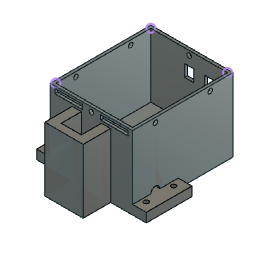
CircuitEnclosure (Autodesk Fusion 360 design; units mm, degrees)
Autodesk Fusion 360 part; units mm, degrees
sketch "Sketch1" plane through (0, 0, 0) normal (0, 1, 0) x (1, 0, 0)
  line L0 (0, 0) -> (60, 0)
  line L1 (60, 0) -> (-60, 0)
  line L2 (-60, 0) -> (-60, -50)
  line L3 (-60, -50) -> (60, -50)
  line L4 (60, -50) -> (60, 0)
  line L5 (-60, 0) -> (-45, 0)
  line L6 (60, 0) -> (45, 0)
  line L7 (-45, 0) -> (-45, 60)
  line L8 (45, 0) -> (45, 60)
  line L9 (-45, 60) -> (45, 60)
  dimension "d1" = 60
  dimension "d2" = 120
  dimension "d3" = 50
  dimension "d4" = 15
  dimension "d5" = 15
  dimension "d6" = 60
  dimension "d7" = 60
  constraint coincident L0.start origin
  constraint horizontal L0
  constraint parallel L0 L1
  constraint perpendicular L1 L2
  constraint perpendicular L2 L3
  constraint perpendicular L1 L4
  constraint perpendicular L2 L5
  constraint perpendicular L4 L6
  constraint perpendicular L5 L7
  constraint perpendicular L6 L8
  measures "d1" distance of L0.start L0.end
  measures "d2" distance of L0.end L1.end
  measures "d3" distance of L1.end L2.end
  measures "d4" distance of L1.end L5.end
  measures "d5" distance of L0.end L6.end
  measures "d6" distance of L5.end L7.end
  measures "d7" distance of L6.end L8.end
extrude "Extrude1" add sketch "Sketch1" along normal blind 10
sketch "Sketch2" plane through (0, 10, 0) normal (0, 1, 0) x (-1, 0, 0)
  line L0 (60, 0) -> (60, 50)
  line L1 (60, 50) -> (-60, 50)
  line L2 (-60, 50) -> (-60, 0)
  line L3 (-60, 0) -> (-45, 0)
  line L4 (-45, 0) -> (-45, -60)
  line L5 (-45, -60) -> (45, -60)
  line L6 (45, -60) -> (45, 0)
  line L7 (45, 0) -> (60, 0)
  line L8 (60, 50) -> (60, 40)
  line L9 (-60, 50) -> (-60, 40)
  circle A0 centre (50, 40) radius 2.5
  circle A1 centre (-50, 40) radius 2.5
  circle A2 centre (50, 10) radius 2.5
  circle A3 centre (-50, 10) radius 2.5
  dimension "d10" = 10
  dimension "d11" = 10
  dimension "d12" = 10
  dimension "d13" = 10
  dimension "d14" = 5
  dimension "d15" = 5
  dimension "d16" = 30
  dimension "d17" = 5
  dimension "d18" = 30
  dimension "d19" = 5
  constraint coincident L0.end L1.start
  constraint perpendicular L1 L8
  constraint coincident L1.end L2.start
  constraint perpendicular L1 L9
  measures "d10" distance of L0.end L8.end
  measures "d11" distance of L8.end A0.centre
  measures "d12" distance of L1.end L9.end
  measures "d13" distance of L9.end A1.centre
  measures "d14" diameter of A0
  measures "d15" diameter of A1
  measures "d16" distance of A0.centre A2.centre
  measures "d17" diameter of A2
  measures "d18" distance of A1.centre A3.centre
  measures "d19" diameter of A3
extrude "Extrude2" cut sketch "Sketch2" against normal blind 20 contours A0 | A1 | A2 | A3
sketch "Sketch3" plane through (0, 10, 0) normal (0, 1, 0) x (-1, 0, 0)
  circle A0 centre (50, 40) radius 2.5
  circle A1 centre (-50, 40) radius 2.5
  circle A2 centre (50, 10) radius 2.5
  circle A3 centre (-50, 10) radius 2.5
  line L0 (60, 0) -> (60, 50)
  line L1 (60, 50) -> (-60, 50)
  line L2 (-60, 50) -> (-60, 0)
  line L3 (-60, 0) -> (-45, 0)
  line L4 (-45, 0) -> (-45, -60)
  line L5 (-45, -60) -> (45, -60)
  line L6 (45, -60) -> (45, 0)
  line L7 (45, 0) -> (60, 0)
  line L8 (45, -60) -> (45, 50)
  line L9 (-45, -60) -> (-45, 50)
  line L10 (45, 50) -> (-45, 50)
  line L11 (-45, -60) -> (45, -60)
  line L12 (45, 50) -> (42, 50)
  line L13 (45, -60) -> (42, -60)
  line L14 (-45, -60) -> (-45, -57)
  line L15 (-45, 50) -> (-42, 50)
  line L16 (42, 47) -> (42, -57)
  line L17 (-42, -57) -> (42, -57)
  line L18 (-42, -57) -> (-42, 47)
  line L19 (-42, 47) -> (42, 47)
  dimension "d22" = 3
  dimension "d23" = 3
  dimension "d24" = 3
  dimension "d25" = 3
  dimension "d26" = 3
  dimension "d27" = 3
  dimension "d28" = 3
  dimension "d29" = 3
  constraint coincident L5.end L6.start
  constraint coincident L1 L8.end
  constraint perpendicular L1 L8
  constraint coincident L4.end L5.start
  constraint coincident L1 L9.end
  constraint perpendicular L1 L9
  constraint perpendicular L8 L12
  constraint perpendicular L6 L13
  constraint perpendicular L11 L14
  constraint perpendicular L9 L15
  measures "d22" distance of L8.end L12.end
  measures "d23" distance of L12.end L16.start
  measures "d24" distance of L5.end L13.end
  measures "d25" distance of L13.end L16.end
  measures "d26" distance of L4.end L14.end
  measures "d27" distance of L14.end L17.start
  measures "d28" distance of L9.end L15.end
  measures "d29" distance of L15.end L18.end
extrude "Extrude3" add sketch "Sketch3" along normal blind 70 contours L1 L4 L5 L6 L8 L9 L10 L11 L12 L13 L14 L15
sketch "Sketch4" plane through (-45, 0, 0) normal (-1, 0, 0) x (0, 0, 1)
  line L0 (-60, 0) -> (0, 0)
  line L1 (0, 0) -> (0, 10)
  line L2 (0, 10) -> (50, 10)
  line L3 (50, 10) -> (50, 80)
  line L4 (50, 80) -> (-60, 80)
  line L5 (-60, 80) -> (-60, 0)
  line L6 (-60, 80) -> (-60, 75)
  circle A0 centre (-35, 75) radius 2.5
  circle A1 centre (25, 75) radius 2.5
  dimension "d32" = 25
  dimension "d34" = 5
  dimension "d35" = 5
  constraint coincident L4.end L5.start
  constraint coincident L5 L6.end
  constraint perpendicular L4 L6
  measures "d32" distance of L6.end A0.centre
  measures "d34" diameter of A0
  measures "d35" diameter of A1
extrude "Extrude4" cut sketch "Sketch4" against normal blind 10 contours A0 | A1
sketch "Sketch5" plane through (45, 0, 0) normal (1, 0, 0) x (0, 0, -1)
  line L0 (0, 0) -> (60, 0)
  line L1 (60, 0) -> (60, 80)
  line L2 (60, 80) -> (-50, 80)
  line L3 (-50, 80) -> (-50, 10)
  line L4 (-50, 10) -> (0, 10)
  line L5 (0, 10) -> (0, 0)
  line L6 (-50, 80) -> (-50, 75)
  circle A0 centre (-25, 75) radius 2.5
  circle A1 centre (35, 75) radius 2.5
  dimension "d38" = 5
  dimension "d39" = 25
  dimension "d41" = 5
  dimension "d42" = 5
  constraint coincident L2.end L3.start
  constraint perpendicular L2 L6
  measures "d38" distance of L2.end L6.end
  measures "d39" distance of L6.end A0.centre
  measures "d41" diameter of A0
  measures "d42" diameter of A1
extrude "Extrude5" cut sketch "Sketch5" against normal blind 11 contours A0 | A1
sketch "Sketch6" plane through (0, 0, 50) normal (0, 0, 1) x (1, 0, 0)
  line L0 (-60, 0) -> (60, 0)
  line L1 (60, 0) -> (60, 10)
  line L2 (60, 10) -> (45, 10)
  line L3 (45, 10) -> (45, 80)
  line L4 (45, 80) -> (-45, 80)
  line L5 (-45, 80) -> (-45, 10)
  line L6 (-45, 10) -> (-60, 10)
  line L7 (-60, 10) -> (-60, 0)
  circle A0 centre (0, 75) radius 2.5
  dimension "d47" = 5
  measures "d47" diameter of A0
extrude "Extrude6" cut sketch "Sketch6" against normal blind 11 contours A0
sketch "Sketch7" plane through (0, 0, -60) normal (0, 0, -1) x (-1, 0, 0)
  line L0 (-45, 0) -> (45, 0)
  line L1 (45, 0) -> (45, 80)
  line L2 (45, 80) -> (-45, 80)
  line L3 (-45, 80) -> (-45, 0)
  circle A0 centre (0, 75) radius 2.5
  dimension "d51" = 5
  measures "d51" diameter of A0
extrude "Extrude7" cut sketch "Sketch7" against normal blind 11 contours A0
sketch "Sketch8" plane through (0, 0, 50) normal (0, 0, 1) x (1, 0, 0)
  circle A0 centre (0, 75) radius 2.5
  line L0 (-60, 0) -> (60, 0)
  line L1 (60, 0) -> (60, 10)
  line L2 (60, 10) -> (45, 10)
  line L3 (45, 10) -> (45, 80)
  line L4 (45, 80) -> (-45, 80)
  line L5 (-45, 80) -> (-45, 10)
  line L6 (-45, 10) -> (-60, 10)
  line L7 (-60, 10) -> (-60, 0)
  line L8 (-45, 80) -> (-45, 75)
  line L9 (-15, 77.5) -> (-35, 77.5)
  line L10 (-35, 72.5) -> (-15, 72.5)
  line L11 (-15, 77.5) -> (-10, 77.5)
  line L12 (-10, 77.5) -> (-10, 72.5)
  line L13 (-10, 72.5) -> (-15, 72.5)
  line L14 (-35, 77.5) -> (-40, 77.5)
  line L15 (-40, 77.5) -> (-40, 72.5)
  line L16 (-40, 72.5) -> (-35, 72.5)
  dimension "d55" = 20
  dimension "d56" = 5
  dimension "d57" = 5
  constraint coincident L4.end L5.start
  constraint coincident L5 L8.end
  constraint perpendicular L4 L8
  constraint perpendicular L11 L12
  constraint perpendicular L14 L15
  measures "d55" distance of L9.start L9.end
  measures "d56" distance of L9.end L10.start
  measures "d57" distance of L11.end L12.end
extrude "Extrude8" cut sketch "Sketch8" against normal blind 20 contours L9 L10 L11 L12 L13 L14 L15 L16
sketch "Sketch9" plane through (0, 0, 50) normal (0, 0, 1) x (1, 0, 0)
  line L0 (-40, 72.5) -> (-40, 77.5)
  line L1 (-40, 77.5) -> (-10, 77.5)
  line L2 (-10, 77.5) -> (-10, 72.5)
  line L3 (-10, 72.5) -> (-40, 72.5)
  circle A0 centre (0, 75) radius 2.5
  line L4 (-60, 0) -> (60, 0)
  line L5 (60, 0) -> (60, 10)
  line L6 (60, 10) -> (45, 10)
  line L7 (45, 10) -> (45, 80)
  line L8 (45, 80) -> (-45, 80)
  line L9 (-45, 80) -> (-45, 10)
  line L10 (-45, 10) -> (-60, 10)
  line L11 (-60, 10) -> (-60, 0)
  line L12 (45, 80) -> (45, 75)
  line L13 (45, 75) -> (40, 75)
  line L14 (40, 75) -> (40, 72.5)
  line L15 (40, 75) -> (40, 77.5)
  line L16 (40, 77.5) -> (10, 77.5)
  line L17 (10, 77.5) -> (10, 72.5)
  line L18 (10, 72.5) -> (40, 72.5)
  dimension "d60" = 2.5
  dimension "d61" = 2.5
  dimension "d62" = 30
  dimension "d63" = 5
  constraint coincident L7.end L8.start
  constraint coincident L7 L12.end
  constraint perpendicular L8 L12
  constraint perpendicular L12 L13
  constraint perpendicular L13 L14
  constraint perpendicular L13 L15
  constraint perpendicular L15 L16
  constraint perpendicular L16 L17
  measures "d60" distance of L13.end L14.end
  measures "d61" distance of L13.end L15.end
  measures "d62" distance of L15.end L16.end
  measures "d63" distance of L16.end L17.end
extrude "Extrude9" cut sketch "Sketch9" against normal blind 20 contours L14 L15 L16 L17 L18
sketch "Sketch10" plane through (0, 0, 0) normal (0, -1, 0) x (1, 0, 0)
  circle A0 centre (-50, 40) radius 2.5
  circle A1 centre (50, 40) radius 2.5
  circle A2 centre (-50, 10) radius 2.5
  circle A3 centre (50, 10) radius 2.5
  line L0 (-60, 50) -> (-60, 0)
  line L1 (-60, 0) -> (-45, 0)
  line L2 (-45, 0) -> (-45, -60)
  line L3 (-45, -60) -> (45, -60)
  line L4 (45, -60) -> (45, 0)
  line L5 (45, 0) -> (60, 0)
  line L6 (60, 0) -> (60, 50)
  line L7 (60, 50) -> (-60, 50)
  line L8 (0, 50) -> (11, 50)
  line L9 (11, 50) -> (11, 72)
  line L10 (11, 72) -> (-11, 72)
  line L11 (-11, 72) -> (-11, 50)
  line L12 (-11, 50) -> (-21, 50)
  line L13 (-21, 50) -> (-21, 80)
  line L14 (-21, 80) -> (21, 80)
  line L15 (21, 80) -> (21, 50)
  dimension "d66" = 11
  dimension "d67" = 22
  dimension "d68" = 22
  dimension "d69" = 10
  constraint midpoint L7 L8.start
  constraint parallel L7 L8
  constraint perpendicular L8 L9
  constraint perpendicular L9 L10
  constraint coincident L7 L11.end
  constraint perpendicular L7 L11
  constraint perpendicular L11 L12
  constraint perpendicular L7 L13
  constraint perpendicular L13 L14
  constraint coincident L7 L15.end
  constraint perpendicular L7 L15
  measures "d66" distance of L8.start L8.end
  measures "d67" distance of L8.end L9.end
  measures "d68" distance of L9.end L10.end
  measures "d69" distance of L11.end L12.end
extrude "Extrude10" add sketch "Sketch10" against normal blind 70 contours L7 L9 L10 L11 L12 L13 L14 L15
sketch "Sketch11" plane through (0, 0, 0) normal (0, -1, 0) x (1, 0, 0)
  line L0 (-21, 50) -> (-60, 50)
  line L1 (-60, 50) -> (-60, 0)
  line L2 (-60, 0) -> (-45, 0)
  line L3 (-45, 0) -> (-45, -60)
  line L4 (-45, -60) -> (45, -60)
  line L5 (45, -60) -> (45, 0)
  line L6 (45, 0) -> (60, 0)
  line L7 (60, 0) -> (60, 50)
  line L8 (60, 50) -> (21, 50)
  line L9 (21, 50) -> (21, 80)
  line L10 (21, 80) -> (-21, 80)
  line L11 (-21, 80) -> (-21, 50)
  circle A0 centre (-50, 40) radius 2.5
  circle A1 centre (50, 40) radius 2.5
  circle A2 centre (-50, 10) radius 2.5
  circle A3 centre (50, 10) radius 2.5
  line L12 (-11, 50) -> (-11, 72)
  line L13 (-11, 72) -> (11, 72)
  line L14 (11, 72) -> (11, 50)
  line L15 (11, 50) -> (-11, 50)
sketch "Sketch12" plane through (0, 0, 0) normal (0, -1, 0) x (1, 0, 0)
sketch "Sketch13" plane through (0, 0, 80) normal (0, 0, 1) x (1, 0, 0)
  line L0 (-21, 0) -> (21, 0)
  line L1 (21, 0) -> (21, 70)
  line L2 (21, 70) -> (-21, 70)
  line L3 (-21, 70) -> (-21, 0)
sketch "Sketch14" plane through (-45, 0, 0) normal (-1, 0, 0) x (0, 0, 1)
  circle A0 centre (25, 75) radius 2.5
  circle A1 centre (-35, 75) radius 2.5
  line L0 (-60, 0) -> (0, 0)
  line L1 (0, 0) -> (0, 10)
  line L2 (0, 10) -> (50, 10)
  line L3 (50, 10) -> (50, 80)
  line L4 (50, 80) -> (-60, 80)
  line L5 (-60, 80) -> (-60, 0)
  line L6 (0, 10) -> (25, 10)
  arc A2 (30, 10) -> (20, 10) centre (25, 10) ccw
  dimension "d72" = 10
  constraint coincident L1.end L2.start
  constraint midpoint L2 L6.end
  constraint coincident L6.end A2.centre
  constraint coincident L2 A2.end
  constraint coincident L2 A2.start
  measures "d72" diameter of A2
extrude "Extrude11" cut sketch "Sketch14" against normal blind 100 contours L2 L6 A2
sketch "Sketch15" plane through (0, 0, -60) normal (0, 0, -1) x (-1, 0, 0)
  circle A0 centre (0, 75) radius 2.5
  line L0 (-45, 0) -> (45, 0)
  line L1 (45, 0) -> (45, 80)
  line L2 (45, 80) -> (-45, 80)
  line L3 (-45, 80) -> (-45, 0)
  line L4 (-45, 80) -> (-45, 65)
  line L5 (-30, 65) -> (-17, 65)
  line L6 (-30, 65) -> (-30, 47)
  line L7 (-30, 47) -> (-17, 47)
  line L8 (-17, 47) -> (-17, 65)
  dimension "d76" = 13
  dimension "d77" = 18
  dimension "d78" = 13
  constraint coincident L2.end L3.start
  constraint coincident L3 L4.end
  constraint perpendicular L3 L5
  constraint perpendicular L5 L6
  constraint perpendicular L6 L7
  measures "d76" distance of L5.start L5.end
  measures "d77" distance of L5.start L6.end
  measures "d78" distance of L6.end L7.end
extrude "Extrude12" cut sketch "Sketch15" against normal blind 20 contours L5 L6 L7 L8
sketch "Sketch16" plane through (0, 0, -60) normal (0, 0, -1) x (-1, 0, 0)
  line L0 (-17, 47) -> (-30, 47)
  line L1 (-30, 47) -> (-30, 65)
  line L2 (-30, 65) -> (-17, 65)
  line L3 (-17, 65) -> (-17, 47)
  circle A0 centre (0, 75) radius 2.5
  line L4 (-45, 0) -> (45, 0)
  line L5 (45, 0) -> (45, 80)
  line L6 (45, 80) -> (-45, 80)
  line L7 (-45, 80) -> (-45, 0)
  line L8 (-5, 65) -> (5, 65)
  line L9 (-5, 65) -> (-5, 52)
  line L10 (-5, 52) -> (5, 52)
  line L11 (5, 52) -> (5, 65)
  dimension "d81" = 10
  dimension "d82" = 13
  dimension "d83" = 10
  constraint perpendicular L3 L8
  constraint perpendicular L8 L9
  constraint perpendicular L9 L10
  measures "d81" distance of L8.start L8.end
  measures "d82" distance of L8.start L9.end
  measures "d83" distance of L9.end L10.end
extrude "Extrude13" cut sketch "Sketch16" against normal blind 20 contours L8 L9 L10 L11
sketch "Sketch17" plane through (0, 80, 0) normal (0, 1, 0) x (-1, 0, 0)
  line L0 (42, -57) -> (-42, -57)
  line L1 (-42, -57) -> (-42, 47)
  line L2 (-42, 47) -> (42, 47)
  line L3 (42, 47) -> (42, -57)
  line L4 (-45, -60) -> (45, -60)
  line L5 (45, -60) -> (45, 50)
  line L6 (45, 50) -> (-45, 50)
  line L7 (-45, 50) -> (-45, -60)
sketch "Sketch18" plane through (0, 0, 50) normal (0, 0, 1) x (1, 0, 0)
  line L0 (-11, 70) -> (-11, 0)
  line L1 (-11, 0) -> (11, 0)
  line L2 (11, 0) -> (11, 70)
  line L3 (11, 70) -> (21, 70)
  line L4 (21, 70) -> (21, 0)
  line L5 (21, 0) -> (60, 0)
  line L6 (60, 0) -> (60, 10)
  line L7 (60, 10) -> (45, 10)
  line L8 (45, 10) -> (45, 80)
  line L9 (45, 80) -> (-45, 80)
  line L10 (-45, 80) -> (-45, 10)
  line L11 (-45, 10) -> (-60, 10)
  line L12 (-60, 10) -> (-60, 0)
  line L13 (-60, 0) -> (-21, 0)
  line L14 (-21, 0) -> (-21, 70)
  line L15 (-21, 70) -> (-11, 70)
  line L16 (10, 77.5) -> (40, 77.5)
  line L17 (40, 77.5) -> (40, 72.5)
  line L18 (40, 72.5) -> (10, 72.5)
  line L19 (10, 72.5) -> (10, 77.5)
  line L20 (-40, 72.5) -> (-40, 77.5)
  line L21 (-40, 77.5) -> (-10, 77.5)
  line L22 (-10, 77.5) -> (-10, 72.5)
  line L23 (-10, 72.5) -> (-40, 72.5)
  circle A0 centre (0, 75) radius 2.5
sketch "Sketch19" plane through (0, 80, 0) normal (0, 1, 0) x (-1, 0, 0)
sketch "Sketch20" plane through (0, 0, 50) normal (0, 0, 1) x (1, 0, 0)
sketch "Sketch21" plane through (-45, 0, 0) normal (-1, 0, 0) x (0, 0, 1)
  arc A0 (30, 10) -> (20, 10) centre (25, 10) ccw
  line L0 (30, 10) -> (50, 10)
  line L1 (50, 10) -> (50, 80)
  line L2 (50, 80) -> (-60, 80)
  line L3 (-60, 80) -> (-60, 0)
  line L4 (-60, 0) -> (0, 0)
  line L5 (0, 0) -> (0, 10)
  line L6 (0, 10) -> (20, 10)
  circle A1 centre (-35, 75) radius 2.5
  circle A2 centre (25, 75) radius 2.5
sketch "Sketch22" plane through (0, 80, 0) normal (0, 1, 0) x (-1, 0, 0)
sketch "Sketch23" plane through (-45, 0, 0) normal (-1, 0, 0) x (0, 0, 1)
sketch "Sketch24" plane through (45, 0, 0) normal (1, 0, 0) x (0, 0, -1)
  arc A0 (-20, 10) -> (-30, 10) centre (-25, 10) ccw
  line L0 (-20, 10) -> (0, 10)
  line L1 (0, 10) -> (0, 0)
  line L2 (0, 0) -> (60, 0)
  line L3 (60, 0) -> (60, 80)
  line L4 (60, 80) -> (-50, 80)
  line L5 (-50, 80) -> (-50, 10)
  line L6 (-50, 10) -> (-30, 10)
  circle A1 centre (35, 75) radius 2.5
  circle A2 centre (-25, 75) radius 2.5
sketch "Sketch25" plane through (0, 80, 0) normal (0, 1, 0) x (-1, 0, 0)
  point P0 (42, -57)
  point P1 (-42, -57)
  point P2 (42, 47)
  dimension "d86" = 84
  dimension "d87" = 104
  measures "d86" distance of P0 P1
  measures "d87" distance of P0 P2
